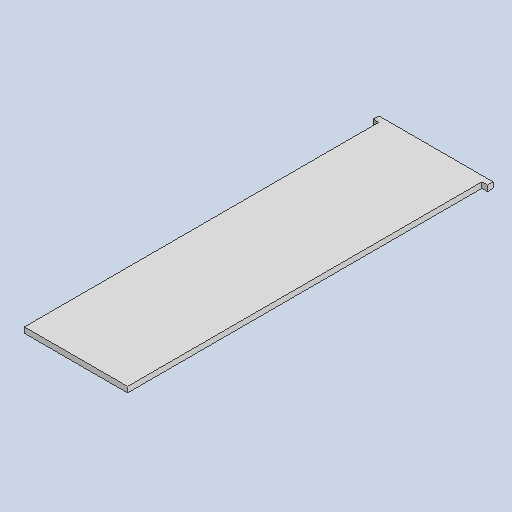
# Autodesk Inventor part: wall 2 for sorting
Saved by Autodesk Inventor 2025.3 (Build 293356000, 356)
## iProperties
Created: 2026-05-24
Part Number: wall 2 for sorting
Material: Generic
Document SubType Name: Modeling
Designer: kamal
Density: 1 g/cm^3
Appearance: Default
Author: kamal
Autodesk Inventor part; units mm, degrees
ref_plane "YZ Plane" through (0, 0, 0) normal (1, 0, 0) x (0, 1, 0)
ref_plane "XZ Plane" through (0, 0, 0) normal (0, 1, 0) x (-1, 0, 0)
ref_plane "XY Plane" through (0, 0, 0) normal (0, 0, 1) x (1, 0, 0)
sketch "Sketch1" plane through (0, 0, 0) normal (0, 1, 0) x (-1, 0, 0)
  line L0 (0, 0) -> (6, 0)
  line L1 (6, 0) -> (6, -6)
  line L2 (6, -6) -> (0, -6)
  line L3 (0, -6) -> (0, 0)
  line L4 (0, -6) -> (-55, -6)
  line L5 (-55, -6) -> (-55, 378)
  line L6 (-55, 378) -> (0, 378)
  line L7 (0, 378) -> (0, -6)
  dimension "d0" = 6
  dimension "d1" = 6
  dimension "d2" = 55
  dimension "d3" = 384
  constraints: 16 end point, 4 parallel, 2 horizontal, 2 perpendicular
  measures "d0" distance of L1.end L2.end
  measures "d1" distance of L0.end L1.end
  measures "d2" distance of L5.end L6.end
  measures "d3" distance of L4.end L5.end
extrude "Extrusion1" add sketch "Sketch1" along normal blind 6
mirror "Mirror1" about plane through (55, 0, 378) normal (1, 0, 0) of "Extrusion1"
body "Solid1"
